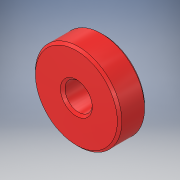
# Autodesk Inventor part: ベアリング_6-19-6
Saved by Autodesk Inventor 2019.4 (Build 234330000, 330)
## iProperties
Created: 2021-12-04
Part Number: ベアリング_6-19-6
Material: 一般
Document SubType Name: Modeling
Designer: 堀川皓史
Density: 1 g/cm^3
Appearance: 淡い赤
Author: 堀川皓史
Autodesk Inventor part; units mm, degrees
ref_plane "YZ Plane" through (0, 0, 0) normal (1, 0, 0) x (0, 1, 0)
ref_plane "XZ Plane" through (0, 0, 0) normal (0, 1, 0) x (-1, 0, 0)
ref_plane "XY Plane" through (0, 0, 0) normal (0, 0, 1) x (1, 0, 0)
sketch "スケッチ1" plane through (0, 0, 0) normal (0, 0, 1) x (1, 0, 0)
  circle A0 centre (0, 0) radius 3
  circle A1 centre (0, 0) radius 9.5
  dimension "d0" = 6
  dimension "d1" = 19
  constraints: 2 centre point, 2 coincident
  measures "d0" diameter of A0
  measures "d1" diameter of A1
extrude "押し出し1" add sketch "スケッチ1" along normal blind 6
chamfer "面取り1" distance 0.5 angle 45 4 edges at (-9.5, 0, 6) (-9.5, 0, 0) (-3, 0, 6) (-3, 0, 0)
